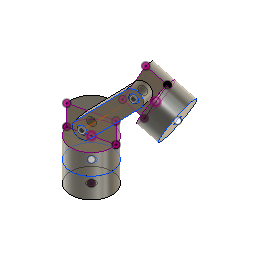
Day16 - Robotic arm part1 (Autodesk Fusion 360 design; units mm, degrees)
Autodesk Fusion 360 part; units mm, degrees
sketch "Sketch1" plane through (0, 0, 0) normal (0, 0, 1) x (1, 0, 0) in component "Component"
  circle A0 centre (0, 0) radius 50
  circle A1 centre (0, 0) radius 10
  dimension "d1" = 100
  dimension "d2" = 20
  measures "d1" diameter of A0
  measures "d2" diameter of A1
extrude "Extrude1" add sketch "Sketch1" along normal blind 50 contours A0 | A1 makes body 1 in component "Component"
extrude "Extrude2" add sketch "Sketch1" along normal blind 30 from surface at 50 contours A1 bodies 1 in component "Component"
sketch "Sketch1 (2)" plane through (0, 0, 0) normal (0, 0, 1) x (1, 0, 0) in component "Component'"
  circle A0 centre (-214.7924, -0.6712) radius 50
  circle A1 centre (-214.7924, -0.6712) radius 10
  dimension "d8" = 100
  dimension "d9" = 20
  measures "d8" diameter of A0
  measures "d9" diameter of A1
extrude "Extrude1'" add sketch "Sketch1 (2)" along normal blind 50 separate body makes body 2 in component "Component'"
extrude "Extrude2'" add sketch "Sketch1 (2)" along normal up to surface (20 mm away) from surface at 30 contours A1 bodies 2 in component "Component'"
sketch "Sketch2" plane through (0, 0, 50) normal (0, 0, 1) x (-1, 0, 0) in component "Component'"
  circle A0 centre (214.7924, 0.6712) radius 50
  line L0 (264.7924, 0.6712) -> (164.7924, 0.6712)
extrude "Extrude3" add sketch "Sketch2" along normal blind 50 contours A0 L0 picked at (207.1995, -18.6751) bodies 2 in component "Component'"
sketch "Sketch3" plane through (0, -0.6712, 0) normal (0, -1, 0) x (1, 0, 0) in component "Component'"
  line L0 (-264.7924, 50) -> (-164.7924, 50)
  line L1 (-164.7924, 50) -> (-164.7924, 100)
  line L2 (-164.7924, 100) -> (-264.7924, 100)
  line L3 (-264.7924, 100) -> (-264.7924, 50)
  circle A0 centre (-214.7924, 80) radius 10
  dimension "d17" = 20
  dimension "d18" = 20
  measures "d17" diameter of A0
extrude "Extrude4" add sketch "Sketch3" along normal blind 30 contours A0 bodies 2 in component "Component'"
sketch "Sketch1 (3)" plane through (0, 0, 50) normal (0, 0, 1) x (-1, 0, 0) in component "Component''"
  line L0 (527.8882, 20.1997) -> (379.5594, 20.1997)
  arc A0 (379.5594, 20.1997) -> (379.5594, -19.8003) centre (379.5594, 0.1997) ccw
  line L1 (379.5594, -19.8003) -> (527.8882, -19.8003)
  arc A1 (527.8882, -19.8003) -> (527.8882, 20.1997) centre (527.8882, 0.1997) ccw
  line L2 (527.8882, 0.1997) -> (379.5594, 0.1997) construction
  circle A2 centre (527.8882, 0.1997) radius 10
  circle A3 centre (379.5594, 0.1997) radius 10
  dimension "d21" = 20
  dimension "d23" = 10
  measures "d21" diameter of A2
  measures "d23" distance of A0 A3
extrude "Extrude1''" add sketch "Sketch1 (3)" along normal blind 30 separate body makes body 3 in component "Component''"
sketch "Sketch1 (4)" plane through (0, 0, 0) normal (0, 0, 1) x (1, 0, 0) in component "Component'''"
  circle A0 centre (-221.7811, 2.1941) radius 50
  circle A1 centre (-221.7811, 2.1941) radius 10
  dimension "d8_1" = 100
  dimension "d9_1" = 20
  measures "d8_1" diameter of A0
  measures "d9_1" diameter of A1
extrude "Extrude1'''" add sketch "Sketch1 (4)" along normal blind 50 separate body makes body 4 in component "Component'''"
extrude "Extrude2''" add sketch "Sketch1 (4)" along normal up to surface (20 mm away) from surface at 30 contours A1 bodies 4 in component "Component'''"
sketch "Sketch2 (2)" plane through (0, 0, 50) normal (0, 0, 1) x (-1, 0, 0) in component "Component'''"
  circle A0 centre (221.7811, -2.1941) radius 50
  line L0 (271.7811, -2.1941) -> (171.7811, -2.1941)
extrude "Extrude3'" add sketch "Sketch2 (2)" along normal blind 50 contours A0 L0 picked at (234.7391, -18.4429) bodies 4 in component "Component'''"
sketch "Sketch3 (2)" plane through (0, 2.1941, 0) normal (0, -1, 0) x (1, 0, 0) in component "Component'''"
  line L0 (-271.7811, 50) -> (-171.7811, 50)
  line L1 (-171.7811, 50) -> (-171.7811, 100)
  line L2 (-171.7811, 100) -> (-271.7811, 100)
  line L3 (-271.7811, 100) -> (-271.7811, 50)
  circle A0 centre (-221.7811, 80) radius 10
  dimension "d17_1" = 20
  dimension "d18_1" = 20
  measures "d17_1" diameter of A0
extrude "Extrude4'" add sketch "Sketch3 (2)" along normal blind 30 contours A0 bodies 4 in component "Component'''"
component "Component" placed x (1, 0, 0) y (0, 1, 0) z (0, 0, 1) at (0, 0, 0)
component "Component'" placed x (1, 0, 0) y (0, 1, 0) z (0, 0, 1) at (214.7924, 0.6712, 50)
component "Component''" placed x (1, 0, 0) y (0, 0, -1) z (0, 1, 0) at (379.5594, -80, 129.8003)
component "Component'''" placed x (1, 0, 0) y (0, 1, 0) z (0, 0, 1) at (73.4522, -2.1941, 50)
